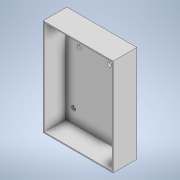
# Autodesk Inventor part: case
Saved by Autodesk Inventor 2020 (Build 240168000, 168)
## iProperties
Created: 2020-04-03
Part Number: case
Material: 일반
Document SubType Name: Modeling
Designer: orphe
Density: 1 g/cm^3
Appearance: 기본값
Author: orphe
Autodesk Inventor part; units mm, degrees
ref_plane "YZ Plane" through (0, 0, 0) normal (1, 0, 0) x (0, 1, 0)
ref_plane "XZ Plane" through (0, 0, 0) normal (0, 1, 0) x (-1, 0, 0)
ref_plane "XY Plane" through (0, 0, 0) normal (0, 0, 1) x (1, 0, 0)
sketch "스케치1" plane through (0, 0, 0) normal (0, 0, 1) x (1, 0, 0)
  line L0 (-32.5, 45) -> (32.5, 45)
  line L1 (32.5, 45) -> (32.5, -45)
  line L2 (32.5, -45) -> (-32.5, -45)
  line L3 (-32.5, -45) -> (-32.5, 45)
  line L4 (-32.5, 45) -> (32.5, -45) construction
  line L5 (32.5, 45) -> (-32.5, -45) construction
  point P0 (0, 0)
  dimension "d1" = 65
  dimension "d2" = 90
  constraints: 12 end point, 2 midpoint, 2 parallel, 1 horizontal, 1 perpendicular
  measures "d1" distance of L1.end L2.end
  measures "d2" distance of L0.end L1.end
extrude "돌출1" add sketch "스케치1" along normal blind 2
sketch "스케치2" plane through (0, 0, 2) normal (0, 0, 1) x (1, 0, 0)
  circle A0 centre (-24, -31) radius 2
  line L0 (-32.5, -45) -> (32.5, -45) projected
  line L1 (-32.5, 45) -> (-32.5, -45) projected
  circle A1 centre (24, -31) radius 2
  line L2 (32.5, -45) -> (32.5, 45) projected
  circle A2 centre (-19, 20.5) radius 2
  circle A3 centre (9, 20.5) radius 2
  point P0 (0, 0)
  dimension "d14" = 4
  dimension "d15" = 14
  dimension "d16" = 8.5
  dimension "d17" = 4
  dimension "d18" = 14
  dimension "d19" = 8.5
  dimension "d20" = 4
  dimension "d21" = 65.5
  dimension "d22" = 13.5
  dimension "d23" = 4
  dimension "d24" = 23.5
  dimension "d25" = 65.5
  constraints: 4 centre point
  measures "d14" diameter of A0
  measures "d15" distance from line of L0 A0.centre
  measures "d16" distance from line of L1 A0.centre
  measures "d17" diameter of A1
  measures "d18" distance from line of L0 A1.centre
  measures "d19" distance from line of L2 A1.centre
  measures "d20" diameter of A2
  measures "d21" distance from line of L0 A2.centre
  measures "d22" distance from line of L1 A2.centre
  measures "d23" diameter of A3
  measures "d24" distance from line of L2 A3.centre
  measures "d25" distance from line of L0 A3.centre
extrude "돌출2" cut sketch "스케치2" against normal blind 2
sketch "스케치3" plane through (0, 0, 2) normal (0, 0, 1) x (1, 0, 0)
  line L0 (32.5, -45) -> (32.5, 45) projected
  line L1 (-32.5, -45) -> (32.5, -45)
  line L2 (32.5, -45) -> (32.5, 45)
  line L3 (32.5, 45) -> (-32.5, 45)
  line L4 (-32.5, 45) -> (-32.5, -45)
  line L5 (-32.5, -45) -> (32.5, 45) construction
  line L6 (32.5, -45) -> (-32.5, 45) construction
  line L7 (-31.5, -44) -> (31.5, -44)
  line L8 (31.5, -44) -> (31.5, 44)
  line L9 (31.5, 44) -> (-31.5, 44)
  line L10 (-31.5, 44) -> (-31.5, -44)
  line L11 (-31.5, -44) -> (31.5, 44) construction
  line L12 (31.5, -44) -> (-31.5, 44) construction
  point P0 (0, 0)
  dimension "d28" = 63
  dimension "d29" = 88
  constraints: 24 end point, 4 midpoint, 4 parallel, 2 horizontal, 2 perpendicular
  measures "d28" distance of L9.end L8.end
  measures "d29" distance of L8.end L7.end
extrude "돌출3" add sketch "스케치3" along normal blind 20
